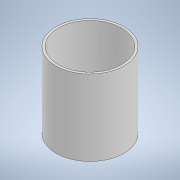
# Autodesk Inventor part: Cylinder_500ml_new
Saved by Autodesk Inventor 2020 (Build 240168000, 168)
## iProperties
Created: 2023-05-12
Part Number: Cylinder_500ml_new
Material: Generic
Document SubType Name: Modeling
Designer: DSOB
Density: 1 g/cm^3
Appearance: Default
Author: DSOB
Autodesk Inventor part; units mm, degrees
ref_plane "YZ Plane" through (0, 0, 0) normal (1, 0, 0) x (0, 1, 0)
ref_plane "XZ Plane" through (0, 0, 0) normal (0, 1, 0) x (-1, 0, 0)
ref_plane "XY Plane" through (0, 0, 0) normal (0, 0, 1) x (1, 0, 0)
sketch "Sketch1" plane through (0, 0, 0) normal (0, 0, 1) x (1, 0, 0)
  line L0 (45, 0) -> (45, 100.2239)
  line L1 (45, 100.2239) -> (42, 100.2239)
  line L2 (42, 100.2239) -> (42, 10)
  line L3 (42, 10) -> (0, 10)
  line L4 (0, 10) -> (0, 0)
  line L5 (0, 0) -> (45, 0)
  line L6 (0, -20.0448) -> (0, 120.2687) projected
  dimension "d1" = 3
  dimension "d8" = 42
  dimension "d10" = 10
  dimension "d11" = 90.2239
  constraints: 12 end point, 4 perpendicular, 1 horizontal
  measures "d1" distance between parallel lines of L0 L2
  measures "d8" distance from line of L4.end L2
  measures "d10" distance between parallel lines of L3 L5
  measures "d11" distance between parallel lines of L3 L1
revolve "Revolution1" add sketch "Sketch1" angle 360 about axis through (0, -10, 0) along (0, 1, 0)
body "Solid1"
